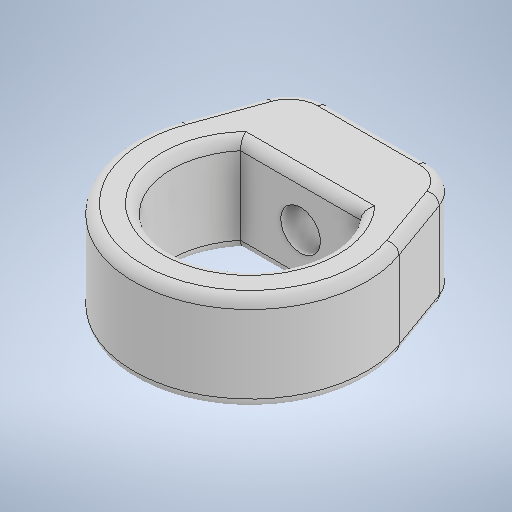
# Autodesk Inventor part: ShaftLock-8mm
Saved by Autodesk Inventor 2025.3 (Build 293356030, 356C)
## iProperties
Created: 2025-10-24
Part Number: ShaftLock-8mm
Material: Generic
Document SubType Name: Modeling
Designer: tvoko
Density: 1 g/cm^3
Appearance: Default
Author: tvoko
Autodesk Inventor part; units mm, degrees
ref_plane "YZ Plane" through (0, 0, 0) normal (1, 0, 0) x (0, 1, 0)
ref_plane "XZ Plane" through (0, 0, 0) normal (0, 1, 0) x (-1, 0, 0)
ref_plane "XY Plane" through (0, 0, 0) normal (0, 0, 1) x (1, 0, 0)
sketch "Sketch1" plane through (0, 0, 0) normal (0, 1, 0) x (-1, 0, 0)
  arc A0 (3.1052, -2.6) -> (-3.1052, -2.6) centre (0, 0) ccw
  line L0 (3.1052, -2.6) -> (-3.1052, -2.6)
  line L1 (0, 0) -> (0, -8.9628) construction
  line L2 (0, -4.05) -> (-4.05, -4.05) construction
  line L3 (-4.05, -4.05) -> (-4.05, 0) construction
  arc A1 (5.6449, -2.0334) -> (-5.6449, -2.0334) centre (0, 0) ccw
  arc A2 (0, -4.05) -> (3.1052, -2.6) centre (0, 0) ccw construction
  arc A3 (-3.1052, -2.6) -> (0, -4.05) centre (0, 0) ccw construction
  line L4 (2.5946, -6.6) -> (-2.5946, -6.6)
  line L5 (4.4763, -5.2778) -> (5.6449, -2.0334)
  line L6 (-4.4763, -5.2778) -> (-5.6449, -2.0334)
  arc A4 (2.5946, -6.6) -> (4.4763, -5.2778) centre (2.5946, -4.6) ccw
  arc A5 (-4.4763, -5.2778) -> (-2.5946, -6.6) centre (-2.5946, -4.6) ccw
  arc A6 (0, -6) -> (5.6449, -2.0334) centre (0, 0) ccw construction
  arc A7 (-5.6449, -2.0334) -> (0, -6) centre (0, 0) ccw construction
  point P0 (4, -6.6)
  point P1 (-4, -6.6)
  point P2 (0, -6.6)
  dimension "d0" = 8.1
  dimension "d1" = 2.6
  dimension "d2" = 12
  dimension "d3" = 4
  dimension "d4" = 8
  dimension "d5" = 2
  constraints: 18 point on circle, 14 end point, 12 tangent, 8 centre point, 7 point on line, 2 coincident, 2 horizontal, 2 perpendicular, 1 equal radius, 1 midpoint, 1 vertical
  measures "d0" diameter of A0
  measures "d1" distance from line of point (0, 0) L0
  measures "d2" diameter of A1
  measures "d3" distance between parallel lines of L0 L4
  measures "d4" distance of point (4, -6.6) point (-4, -6.6)
  measures "d5" radius of A4
extrude "Extrusion1" add sketch "Sketch1" along normal blind 5
sketch "Sketch2" plane through (2.5946, 0, -6.6) normal (0, 0, -1) x (-1, 0, 0)
  line L0 (0, 0) -> (5.1892, 0) projected
  line L1 (5.1892, 0) -> (5.1892, 5) projected
  line L2 (0, 5) -> (5.1892, 5) projected
  line L3 (0, 0) -> (0, 5) projected
  line L4 (5.1892, 2.5) -> (0, 2.5) construction
  line L5 (2.5946, 5) -> (2.5946, 0) construction
  circle A0 centre (2.5946, 2.5) radius 1.025
  dimension "d8" = 2.05
  constraints: 4 end point, 4 midpoint, 1 centre point, 1 vertical
  measures "d8" diameter of A0
extrude "Extrusion2" cut sketch "Sketch2" against normal blind 5 contours A0
fillet "Fillet1" radius 0.5 1 edges at (1.025, 2.5, -6.6)
fillet "Fillet2" radius 0.5 16 edges at (0, 5, 4.05) (0, 0, 4.05) (0, 0, -2.6) (0, 5, -2.6) (0, 0, 6) (5.0606, 0, -3.6556) (3.7445, 0, -6.2364) (0, 0, -6.6) (-3.7445, 0, -6.2364) (-5.0606, 0, -3.6556) (0, 5, -6.6) (-3.7445, 5, -6.2364) (-5.0606, 5, -3.6556) (0, 5, 6) (5.0606, 5, -3.6556) (3.7445, 5, -6.2364)
body "Solid1"
